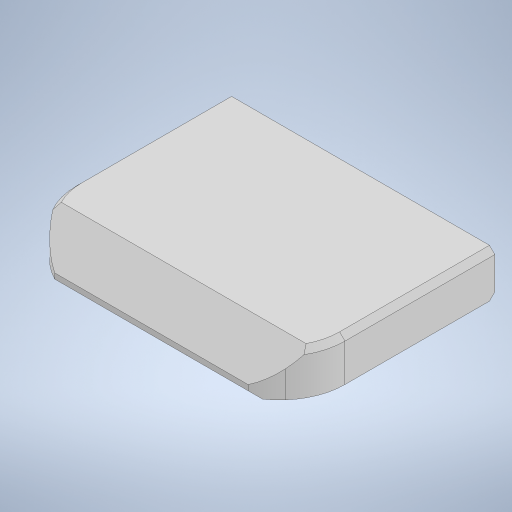
# Autodesk Inventor part: main_body
Saved by Autodesk Inventor 2024.2 (Build 282272000, 272)
## iProperties
Created: 2024-03-07
Part Number: main_body
Material: Ogólny
Document SubType Name: Modeling
Designer: Daniel
Density: 1 g/cm^3
Appearance: Domyślna
Author: Daniel
Autodesk Inventor part; units mm, degrees
ref_plane "YZ Plane" through (0, 0, 0) normal (1, 0, 0) x (0, 1, 0)
ref_plane "XZ Plane" through (0, 0, 0) normal (0, 1, 0) x (-1, 0, 0)
ref_plane "XY Plane" through (0, 0, 0) normal (0, 0, 1) x (1, 0, 0)
sketch "Szkic1" plane through (0, 0, 0) normal (0, 1, 0) x (-1, 0, 0)
  line L0 (-125, 75) -> (124.069178, 75)
  line L1 (125, 64.472311) -> (125, -75)
  line L2 (125, -75) -> (-125, -75)
  line L3 (-125, 75) -> (125, -75) construction
  line L4 (125, 75) -> (-125, -75) construction
  line L5 (-90, 119.581876) -> (90, 119.581876)
  line L6 (0, -118.695088) -> (0, 172.852507) construction
  arc A0 (109.720584, 104.473178) -> (90, 119.581876) centre (60, 60) ccw
  arc A1 (125, 64.472311) -> (109.720584, 104.473178) centre (65, 64.472311) ccw
  line L7 (0, 119.581876) -> (0, -75) construction
  line L8 (-125, 64.472311) -> (-125, -75)
  arc A2 (-90, 119.581876) -> (-109.720584, 104.473178) centre (-60, 60) ccw
  arc A3 (-109.720584, 104.473178) -> (-125, 64.472311) centre (-65, 64.472311) ccw
  point P0 (0, 0)
  point P1 (-124.069178, 75)
  dimension "d0" = 250
  dimension "d1" = 150
  dimension "d9" = 180
  dimension "d10" = 15
  dimension "d11" = 65
  dimension "d29" = 60
  constraints: 18 end point, 10 point on circle, 4 centre point, 4 midpoint, 4 point on line, 4 symmetric about line, 2 horizontal, 2 perpendicular, 2 tangent, 1 equal length, 1 parallel, 1 vertical, 2 other
  measures "d0" distance of L1.end L2.end
  measures "d1" distance of L4.start L1.end
  measures "d9" distance of L5.start L5.end
  measures "d10" distance from line of A0.centre L0
  measures "d11" distance from line of L1 A0.centre
  measures "d29" distance from line of L1 A1.centre
extrude "Wyciągnięcie proste1" add sketch "Szkic1" along normal blind 10
sketch "Szkic3" plane through (0, 10, 0) normal (0, 1, 0) x (1, 0, 0)
  line L0 (125, 75) -> (-125, 75)
  line L1 (-125, 75) -> (-125, -64.472311)
  arc A0 (-109.720584, -104.473178) -> (-90, -119.581876) centre (-60, -60) ccw
  line L2 (-90, -119.581876) -> (90, -119.581876)
  line L3 (95, 45) -> (-95, 45)
  line L4 (-95, 45) -> (-95, -71.068007)
  arc A1 (-95, -71.068007) -> (-81.735072, -89.581876) centre (-60, -60) ccw
  line L5 (-81.735072, -89.581876) -> (81.735072, -89.581876)
  arc A2 (81.735072, -89.581876) -> (95, -71.068007) centre (60, -60) ccw
  line L6 (95, -71.068007) -> (95, 45)
  arc A3 (90, -119.581876) -> (125, -75) centre (60, -60) ccw
  line L7 (125, -75) -> (93.503743, -75)
  line L8 (0, -119.581876) -> (0, 75) construction
  line L9 (-125, -75) -> (-93.503743, -75)
  arc A4 (-125, -64.472311) -> (-109.720584, -104.473178) centre (-65, -64.472311) ccw
  arc A5 (90, -119.581876) -> (109.720584, -104.473178) centre (60, -60) ccw
  arc A6 (109.720584, -104.473178) -> (125, -64.472311) centre (65, -64.472311) ccw
  line L10 (125, -64.472311) -> (125, 75)
  point P0 (124.069178, -75)
  point P1 (-124.069178, -75)
  point P2 (109.720584, -104.473178)
  constraints: 14 end point, 5 point on circle, 2 centre point, 2 midpoint, 1 horizontal, 1 symmetric about line, 3 other
chamfer "Faza2" distance 5 angle 45 4 edges at (0, 0, 119.5819) (-100.5698, 0, 112.9536) (-125, 0, -5.2638) (0, 0, -75)
extrude "Wyciągnięcie proste4" add sketch "Szkic3" along normal blind 30 contours L10 A6 L7 A2 L6 L3 L4 A1 L9 A4 L1 L0 | A2 L5 A1 L4 L3 L6
chamfer "Faza3" distance 30 angle 45 1 edges at (0, 10, 89.5819)
chamfer "Faza4" distance 5 angle 45 4 edges at (-123.6071, 40, 77.3255) (-125, 40, -5.2638) (125, 40, -5.2638) (123.6071, 40, 77.3255)
